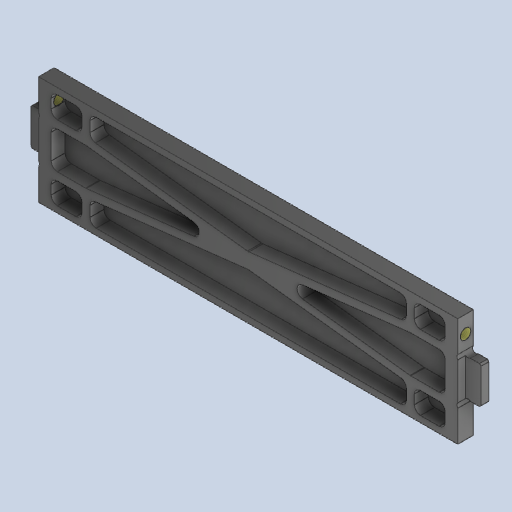
# Autodesk Inventor part: Cockpit_battery_front_frame
Saved by Autodesk Inventor 2022 (Build 260153000, 153)
## iProperties
Part Number: Cockpit_battery_front_frame
Material: アセタール樹脂、黒
Document SubType Name: Modeling
Designer: Masato Kubotera
Density: 1.425 g/cm^3
Appearance: 滑らか - 黒
Description: POM T5
Mass: 13.79 g
Surface Area: 149.623 cm^2
Volume: 9.6772 cm^3
Author: Masato Kubotera
Autodesk Inventor part; units mm, degrees
ref_plane "XZ Plane" through (0, 0, 0) normal (0, 1, 0) x (-1, 0, 0)
derived "Cockpit_side_frame.ipt"
sketch "スケッチ2" plane through (0, 0, 0) normal (0, 1, 0) x (-1, 0, 0)
  line L0 (-23.5, -22.5) -> (-28.5, -27.5)
  line L1 (-28.5, -27.5) -> (-28.5, -91)
  line L2 (-28.5, -91) -> (-23.5, -96)
  line L3 (-23.5, -96) -> (34.25, -96)
  line L4 (36.25, -98) -> (36.25, -131)
  line L5 (36.25, -131) -> (41.25, -136)
  line L6 (41.25, -136) -> (86.5, -136)
  line L7 (91.5, -131) -> (91.5, -20)
  line L8 (91.5, -20) -> (89, -17.5)
  line L9 (89, -17.5) -> (83.25, -17.5)
  line L10 (83.25, -17.5) -> (83.25, -21.0151)
  line L11 (81.7651, -22.5) -> (76.9849, -22.5)
  line L12 (75.5, -21.0151) -> (75.5, -17.5)
  line L13 (75.5, -17.5) -> (67.5, -17.5)
  line L14 (67.5, -17.5) -> (67.5, -21.0151)
  line L15 (66.0151, -22.5) -> (-23.5, -22.5)
  line L16 (-25.25, -25) -> (-20.25, -25) construction
  line L17 (-20.25, -25) -> (-20.25, -93.5) construction
  line L18 (-20.25, -93.5) -> (-25.25, -93.5) construction
  line L19 (-25.25, -93.5) -> (-25.25, -25) construction
  line L20 (-26, -25) -> (-25.25, -25) construction
  line L21 (-25.25, -93.5) -> (-26, -93.5) construction
  line L22 (-26, -93.5) -> (-26, -25) construction
  line L23 (-20.25, -93.5) -> (83.25, -93.5) construction
  line L24 (-20.25, -88.5) -> (83.25, -88.5) construction
  line L25 (83.25, -22.5) -> (83.25, -90.5) construction
  line L26 (83.25, -90.5) -> (88.25, -90.5) construction
  line L27 (88.25, -90.5) -> (88.25, -22.5) construction
  line L28 (83.25, -88.5) -> (83.25, -93.5) construction
  line L29 (83.25, -91) -> (88.25, -91) construction
  line L30 (88.25, -91) -> (88.25, -133.5) construction
  line L31 (83.25, -91) -> (83.25, -133.5) construction
  line L32 (83.25, -133.5) -> (88.25, -133.5) construction
  line L33 (38.75, -133.5) -> (38.75, -128.5) construction
  line L34 (38.75, -128.5) -> (38.75, -93.5) construction
  line L35 (43.75, -93.5) -> (43.75, -128.5) construction
  line L36 (38.75, -128.5) -> (43.75, -128.5) construction
  line L37 (41.25, -128.5) -> (41.25, -93.5) construction
  line L38 (38.75, -128.5) -> (82.1145, -128.5) construction
  line L39 (82.1145, -128.5) -> (82.1145, -133.5) construction
  line L40 (82.1145, -133.5) -> (38.75, -133.5) construction
  line L41 (38.75, -131) -> (82.1145, -131) construction
  line L42 (85.75, -91) -> (85.75, -133.5) construction
  circle A0 centre (85.75, -131) radius 2
  arc A1 (83.25, -128.5) -> (88.25, -128.5) centre (85.75, -131) ccw construction
  line L43 (83.25, -91) -> (-20.25, -91) construction
  line L44 (41.25, -111) -> (43.75, -111) construction
  line L45 (60.4322, -128.5) -> (60.4322, -131) construction
  line L46 (41.2, -115.5651) -> (41.2, -106.4349)
  line L47 (43.8, -107.05) -> (43.8, -114.95)
  line L48 (43.8, -117.05) -> (41.2, -104.95) construction
  line L49 (41.2, -117.05) -> (43.8, -104.95) construction
  line L50 (56.4822, -128.45) -> (64.3822, -128.45)
  line L51 (64.9973, -131.05) -> (55.8672, -131.05)
  line L52 (54.3822, -128.45) -> (66.4822, -131.05) construction
  line L53 (66.4822, -128.45) -> (54.3822, -131.05) construction
  line L54 (41.25, -105) -> (43.75, -105) construction
  line L55 (41.25, -117) -> (43.75, -117) construction
  arc A2 (42.6849, -104.95) -> (41.2, -106.4349) centre (41.9425, -105.6925) ccw
  arc A3 (43.8, -107.05) -> (43.8, -104.95) centre (43.8, -106) ccw
  arc A4 (41.2, -115.5651) -> (42.6849, -117.05) centre (41.9425, -116.3075) ccw
  arc A5 (43.8, -117.05) -> (43.8, -114.95) centre (43.8, -116) ccw
  line L56 (54.4322, -131) -> (54.4322, -128.5) construction
  line L57 (66.4322, -128.5) -> (66.4322, -131) construction
  arc A6 (54.3822, -129.5651) -> (55.8672, -131.05) centre (55.1247, -130.3075) ccw
  arc A7 (56.4822, -128.45) -> (54.3822, -128.45) centre (55.4322, -128.45) ccw
  arc A8 (64.9973, -131.05) -> (66.4822, -129.5651) centre (65.7398, -130.3075) ccw
  arc A9 (66.4822, -128.45) -> (64.3822, -128.45) centre (65.4322, -128.45) ccw
  line L58 (54.3822, -129.5651) -> (54.3822, -128.45)
  line L59 (66.4822, -128.45) -> (66.4822, -129.5651)
  line L60 (42.6849, -104.95) -> (43.8, -104.95)
  line L61 (43.8, -117.05) -> (42.6849, -117.05)
  circle A10 centre (48.4322, -131) radius 1.6
  line L62 (88.25, -22.5) -> (88.25, -17.5) construction
  line L63 (89, -17.5) -> (89, -90.5) construction
  line L64 (89, -90.5) -> (88.25, -90.5) construction
  line L65 (-13.5, -82.5) -> (-13.5, -61)
  arc A11 (-13.5, -82.5) -> (-11.5, -84.5) centre (-11.5, -82.5) ccw
  line L66 (45.5, -84.5) -> (-11.5, -84.5)
  arc A12 (45.5, -84.5) -> (47.5, -82.5) centre (45.5, -82.5) ccw
  line L67 (47.5, -61) -> (47.5, -82.5)
  arc A13 (47.5, -61) -> (45.5, -59) centre (45.5, -61) ccw
  line L68 (-11.5, -59) -> (45.5, -59)
  arc A14 (-11.5, -59) -> (-13.5, -61) centre (-11.5, -61) ccw
  line L69 (31.5, -88.5) -> (31.5, -91) construction
  line L70 (85.75, -22.5) -> (85.75, -90.5) construction
  circle A15 centre (85.75, -34) radius 1.6
  circle A16 centre (85.75, -34) radius 3
  circle A17 centre (85.75, -79) radius 3
  circle A18 centre (85.75, -79) radius 1.6
  line L71 (88.25, -22.5) -> (83.25, -22.5) construction
  arc A19 (88.25, -91) -> (83.25, -91) centre (85.75, -131) ccw construction
  circle A20 centre (48.4322, -131) radius 3
  circle A21 centre (41.25, -99) radius 1.6
  circle A22 centre (41.25, -99) radius 3
  line L72 (6.5, -88.5) -> (6.5, -91) construction
  line L73 (56.5, -88.5) -> (56.5, -91) construction
  line L74 (55.0651, -91.05) -> (7.9349, -91.05)
  line L75 (6.45, -89.5651) -> (6.45, -88.45)
  line L76 (8.55, -88.45) -> (54.45, -88.45)
  line L77 (56.55, -88.45) -> (56.55, -89.5651)
  line L78 (56.55, -91.05) -> (6.45, -88.45) construction
  line L79 (6.45, -91.05) -> (56.55, -88.45) construction
  arc A23 (8.55, -88.45) -> (6.45, -88.45) centre (7.5, -88.45) ccw
  arc A24 (6.45, -89.5651) -> (7.9349, -91.05) centre (7.1925, -90.3075) ccw
  arc A25 (55.0651, -91.05) -> (56.55, -89.5651) centre (55.8075, -90.3075) ccw
  arc A26 (56.55, -88.45) -> (54.45, -88.45) centre (55.5, -88.45) ccw
  line L80 (-20.25, -41) -> (83.25, -41) construction
  line L81 (83.25, -36) -> (-20.25, -36) construction
  line L82 (-20.25, -36) -> (-20.25, -41) construction
  line L83 (-20.25, -38.5) -> (83.25, -38.5) construction
  line L84 (31.5, -41) -> (31.5, -36) construction
  line L85 (55.0651, -35.95) -> (7.9349, -35.95)
  line L86 (7.9349, -41.05) -> (55.0651, -41.05)
  line L87 (56.55, -35.95) -> (6.45, -41.05) construction
  line L88 (6.45, -35.95) -> (55.5877, -40.952) construction
  arc A27 (7.9349, -35.95) -> (6.45, -37.4349) centre (7.1925, -36.6925) ccw
  arc A28 (6.45, -39.5651) -> (7.9349, -41.05) centre (7.1925, -40.3075) ccw
  arc A29 (56.55, -37.4349) -> (55.0651, -35.95) centre (55.8075, -36.6925) ccw
  arc A30 (55.0651, -41.05) -> (56.55, -39.5651) centre (55.8075, -40.3075) ccw
  line L89 (6.5, -41) -> (6.5, -36) construction
  line L90 (56.5, -36) -> (56.5, -41) construction
  line L91 (6.45, -37.4349) -> (6.45, -39.5651)
  line L92 (56.55, -39.5651) -> (56.55, -37.4349)
  circle A31 centre (-1, -38.5) radius 1.6
  circle A32 centre (-1, -38.5) radius 3
  circle A33 centre (64, -38.5) radius 1.6
  circle A34 centre (64, -38.5) radius 3
  line L93 (-25.25, -49.25) -> (-26, -49.25) construction
  line L94 (-25.25, -69.25) -> (-26, -69.25) construction
  line L95 (-26, -59.25) -> (-25.25, -59.25) construction
  line L96 (-22.75, -25) -> (-22.75, -93.5) construction
  arc A35 (66.0151, -22.5) -> (67.5, -21.0151) centre (66.7575, -21.7575) ccw
  arc A36 (75.5, -21.0151) -> (76.9849, -22.5) centre (76.2425, -21.7575) ccw
  line L97 (59.75, -22.5) -> (59.75, -32.5) construction
  line L98 (59.75, -32.5) -> (83.25, -32.5) construction
  line L99 (83.25, -32.5) -> (83.25, -22.5) construction
  line L100 (71.5, -17.5) -> (71.5, -32.5) construction
  line L101 (63.5, -22.5) -> (63.5, -17.5) construction
  line L102 (79.5, -22.5) -> (79.5, -17.5) construction
  circle A37 centre (-22.75, -31.75) radius 1.6
  circle A38 centre (-22.75, -31.75) radius 3
  circle A39 centre (-22.75, -86.75) radius 1.6
  circle A40 centre (-22.75, -86.75) radius 3
  line L103 (67.5, -22.5) -> (75.5, -22.5)
  line L104 (88.25, -17.5) -> (52.5, -17.5) construction
  line L105 (52.5, -17.5) -> (52.5, -22.5) construction
  circle A41 centre (85.75, -98.5) radius 1.475
  circle A42 centre (85.75, -103.5) radius 1.475
  circle A43 centre (85.75, -108.5) radius 1.475
  line L106 (48.25, -93.5) -> (78.75, -93.5)
  line L107 (80.75, -95.5) -> (80.75, -124)
  line L108 (78.75, -126) -> (48.25, -126)
  line L109 (46.25, -124) -> (46.25, -95.5)
  arc A44 (48.25, -93.5) -> (46.25, -95.5) centre (48.25, -95.5) ccw
  arc A45 (46.25, -124) -> (48.25, -126) centre (48.25, -124) ccw
  arc A46 (78.75, -126) -> (80.75, -124) centre (78.75, -124) ccw
  arc A47 (80.75, -95.5) -> (78.75, -93.5) centre (78.75, -95.5) ccw
  arc A48 (36.25, -98) -> (34.25, -96) centre (34.25, -98) ccw
  circle A49 centre (-13.5, -55) radius 1.75
  circle A50 centre (-13.5, -55) radius 2
  line L110 (77.85, -78.65) -> (68.65, -78.65) construction
  line L111 (68.65, -78.65) -> (68.65, -64.85) construction
  line L112 (68.65, -64.85) -> (77.85, -64.85) construction
  line L113 (77.85, -64.85) -> (77.85, -78.65) construction
  line L114 (77.85, -78.65) -> (68.65, -64.85) construction
  line L115 (68.65, -78.65) -> (77.85, -64.85) construction
  line L116 (67.95, -64.2) -> (78.55, -64.2) construction
  line L117 (78.55, -64.2) -> (78.55, -79.3) construction
  line L118 (78.55, -79.3) -> (67.95, -79.3) construction
  line L119 (67.95, -79.3) -> (67.95, -64.2) construction
  line L120 (67.95, -64.2) -> (78.55, -79.3) construction
  line L121 (78.55, -64.2) -> (67.95, -79.3) construction
  line L122 (69.3849, -64.15) -> (77.1151, -64.15)
  line L123 (78.6, -65.6349) -> (78.6, -77.8651)
  line L124 (78.6, -79.35) -> (67.9, -64.15) construction
  line L125 (67.9, -79.35) -> (78.6, -64.15) construction
  line L126 (77.9, -78.7) -> (68.6, -64.8) construction
  line L127 (68.6, -78.7) -> (77.9, -64.8) construction
  arc A51 (69.3849, -64.15) -> (67.9, -65.6349) centre (68.6425, -64.8925) ccw
  arc A52 (70.0849, -64.8) -> (68.6, -66.2849) centre (69.3425, -65.5425) ccw
  line L128 (67.9, -71.75) -> (78.6, -71.75) construction
  line L129 (73.25, -64.15) -> (73.25, -78.7063) construction
  arc A53 (78.6, -65.6349) -> (77.1151, -64.15) centre (77.8575, -64.8925) ccw
  arc A54 (77.9, -66.2849) -> (76.4151, -64.8) centre (77.1575, -65.5425) ccw
  arc A55 (68.6, -77.2151) -> (70.0849, -78.7) centre (69.3425, -77.9575) ccw
  arc A56 (67.9, -77.8651) -> (69.3849, -79.35) centre (68.6425, -78.6075) ccw
  arc A57 (76.4151, -78.7) -> (77.9, -77.2151) centre (77.1575, -77.9575) ccw
  arc A58 (77.1151, -79.35) -> (78.6, -77.8651) centre (77.8575, -78.6075) ccw
  line L130 (70.0849, -64.8) -> (76.4151, -64.8)
  line L131 (77.9, -66.2849) -> (77.9, -77.2151)
  line L132 (67.9, -77.8651) -> (67.9, -65.6349)
  line L133 (68.6, -77.2151) -> (68.6, -66.2849)
  line L134 (76.4151, -78.7) -> (70.0849, -78.7)
  line L135 (77.1151, -79.35) -> (69.3849, -79.35)
  line L136 (-13.5, -71.75) -> (47.5, -71.75) construction
  line L137 (85.75, -56.5) -> (88.25, -56.5) construction
  line L138 (89, -54) -> (88.25, -54) construction
  line L139 (85.7, -69.45) -> (85.7, -43.55)
  line L140 (88.2835, -71.3588) -> (85.7, -41.45) construction
  line L141 (85.7, -71.55) -> (88.3, -41.45) construction
  arc A59 (85.7, -41.45) -> (85.7, -43.55) centre (85.7, -42.5) ccw
  arc A60 (88.3, -42.9349) -> (86.8151, -41.45) centre (87.5575, -42.1925) ccw
  arc A61 (85.7, -69.45) -> (85.7, -71.55) centre (85.7, -70.5) ccw
  arc A62 (86.8151, -71.55) -> (88.3, -70.0651) centre (87.5575, -70.8075) ccw
  line L142 (85.75, -41.5) -> (88.25, -41.5) construction
  line L143 (85.75, -71.5) -> (88.25, -71.5) construction
  arc A63 (89.25, -47.1801) -> (88.3, -46.1348) centre (88.2, -47.1801) ccw
  line L144 (89.25, -47.1801) -> (89.25, -65.8199)
  line L145 (88.25, -46.5) -> (89, -46.5) construction
  line L146 (88.25, -66.5) -> (89, -66.5) construction
  arc A64 (88.3, -66.8652) -> (89.25, -65.8199) centre (88.2, -65.8199) ccw
  line L147 (88.3, -42.9349) -> (88.3, -46.1348)
  line L148 (88.3, -66.8652) -> (88.3, -70.0651)
  line L149 (86.8151, -71.55) -> (85.7, -71.55)
  line L150 (85.7, -41.45) -> (86.8151, -41.45)
  line L151 (86.5, -136) -> (91.5, -131)
  arc A65 (81.7651, -22.5) -> (83.25, -21.0151) centre (82.5075, -21.7575) ccw
  circle A66 centre (85.75, -93.5) radius 2
  circle A67 centre (85.75, -93.5) radius 4 construction
  arc A68 (-24.15, -49.25) -> (-26.25, -49.25) centre (-25.2, -49.25) ccw
  line L152 (-26, -49.25) -> (-26.25, -49.25) construction
  line L153 (-26.25, -49.25) -> (-26.25, -69.25)
  line L154 (-24.15, -49.25) -> (-24.15, -69.25)
  arc A69 (-26.25, -69.25) -> (-24.15, -69.25) centre (-25.2, -69.25) ccw
  point P0 (0, 0)
  point P1 (-25.7227, -96)
  point P2 (-23.5, -22.5)
  point P3 (42.5, -111)
  point P4 (60.4322, -129.75)
  point P5 (31.5, -89.75)
  point P6 (31.5, -38.5)
  point P7 (6.45, -41.05)
  point P8 (52.5, -22)
  point P9 (73.25, -71.75)
  point P10 (73.25, -71.75)
  point P11 (87, -56.5)
  dimension "d1" = 43.75
  dimension "d2" = 5
  dimension "d3" = 2.5
  measures "d1" distance from line of point (0, 0) L35
  measures "d2" distance of L35.end L33.end
  measures "d3" distance of L55.start L55.end
ref_plane "作業平面1" through (-43.75, 0, 0) normal (1, 0, 0) x (0, 1, 0)
sketch "スケッチ3" plane through (-43.75, 0, 0) normal (1, 0, 0) x (0, 1, 0)
  line L0 (-135, -93.5) -> (0, -93.5)
  line L1 (0, -128.5) -> (-135, -128.5)
  line L2 (1.4849, -105) -> (5, -105)
  line L3 (5, -105) -> (5, -117)
  arc A0 (0, -103.5151) -> (1.4849, -105) centre (0.7425, -104.2575) ccw
  line L4 (0, -93.5) -> (0, -103.5151)
  line L5 (-134.9908, -111) -> (0, -111) construction
  line L6 (1.4849, -117) -> (5, -117)
  arc A1 (1.4849, -117) -> (0, -118.4849) centre (0.7425, -117.7425) ccw
  line L7 (0, -128.5) -> (0, -118.4849)
  line L8 (0, -105) -> (0, -117)
  line L9 (0, -118.4849) -> (0, -128.5)
  line L10 (-67.5, -93.5) -> (-67.5, -128.5) construction
  line L11 (-136.4849, -105) -> (-140, -105)
  line L12 (-140, -105) -> (-140, -117)
  arc A2 (-136.4849, -105) -> (-135, -103.5151) centre (-135.7425, -104.2575) ccw
  line L13 (-135, -93.5) -> (-135, -103.5151)
  line L14 (-136.4849, -117) -> (-140, -117)
  arc A3 (-135, -118.4849) -> (-136.4849, -117) centre (-135.7425, -117.7425) ccw
  line L15 (-135, -128.5) -> (-135, -118.4849)
  line L16 (-135, -105) -> (-135, -117)
  line L17 (-135, -118.4849) -> (-135, -128.5)
  line L18 (-12, -119.5) -> (-6, -119.5)
  line L19 (-4, -121.5) -> (-4, -124.5)
  line L20 (-6, -126.5) -> (-12, -126.5)
  line L21 (-14, -124.5) -> (-14, -121.5)
  line L22 (-4, -115) -> (-4, -107)
  line L23 (-67.2707, -113.5132) -> (-18.2707, -119.168)
  line L24 (-16.5, -121.1548) -> (-16.5, -124.5)
  line L25 (-18.5, -126.5) -> (-116.5, -126.5)
  line L26 (-6, -117) -> (-15.135, -117)
  line L27 (-15.3643, -116.9868) -> (-50.0251, -112.9868)
  line L28 (-12, -102.5) -> (-6, -102.5)
  line L29 (-4, -100.5) -> (-4, -97.5)
  line L30 (-6, -95.5) -> (-12, -95.5)
  line L31 (-14, -97.5) -> (-14, -100.5)
  line L32 (-67.2707, -108.4868) -> (-18.2707, -102.832)
  line L33 (-16.5, -100.8452) -> (-16.5, -97.5)
  line L34 (-18.5, -95.5) -> (-116.5, -95.5)
  line L35 (-6, -105) -> (-15.135, -105)
  line L36 (-15.3643, -105.0132) -> (-50.0251, -109.0132)
  line L37 (-67.7293, -113.5132) -> (-116.7293, -119.168)
  line L38 (-118.5, -121.1548) -> (-118.5, -124.5)
  line L39 (-118.5, -100.8452) -> (-118.5, -97.5)
  line L40 (-67.7293, -108.4868) -> (-116.7293, -102.832)
  arc A4 (-6, -126.5) -> (-4, -124.5) centre (-6, -124.5) ccw
  arc A5 (-4, -121.5) -> (-6, -119.5) centre (-6, -121.5) ccw
  arc A6 (-12, -119.5) -> (-14, -121.5) centre (-12, -121.5) ccw
  arc A7 (-14, -124.5) -> (-12, -126.5) centre (-12, -124.5) ccw
  arc A8 (-18.5, -126.5) -> (-16.5, -124.5) centre (-18.5, -124.5) ccw
  arc A9 (-16.5, -121.1548) -> (-18.2707, -119.168) centre (-18.5, -121.1548) ccw
  arc A10 (-67.2707, -113.5132) -> (-67.7293, -113.5132) centre (-67.5, -115.5) ccw
  arc A11 (-116.7293, -119.168) -> (-118.5, -121.1548) centre (-116.5, -121.1548) ccw
  arc A12 (-118.5, -124.5) -> (-116.5, -126.5) centre (-116.5, -124.5) ccw
  arc A13 (-118.5, -100.8452) -> (-116.7293, -102.832) centre (-116.5, -100.8452) ccw
  arc A14 (-116.5, -95.5) -> (-118.5, -97.5) centre (-116.5, -97.5) ccw
  arc A15 (-16.5, -97.5) -> (-18.5, -95.5) centre (-18.5, -97.5) ccw
  arc A16 (-18.2707, -102.832) -> (-16.5, -100.8452) centre (-18.5, -100.8452) ccw
  arc A17 (-67.7293, -108.4868) -> (-67.2707, -108.4868) centre (-67.5, -106.5) ccw
  arc A18 (-50.0251, -109.0132) -> (-50.0251, -112.9868) centre (-49.7958, -111) ccw
  arc A19 (-15.135, -105) -> (-15.3643, -105.0132) centre (-15.135, -107) ccw
  arc A20 (-4, -107) -> (-6, -105) centre (-6, -107) ccw
  arc A21 (-6, -117) -> (-4, -115) centre (-6, -115) ccw
  arc A22 (-15.3643, -116.9868) -> (-15.135, -117) centre (-15.135, -115) ccw
  arc A23 (-14, -100.5) -> (-12, -102.5) centre (-12, -100.5) ccw
  arc A24 (-12, -95.5) -> (-14, -97.5) centre (-12, -97.5) ccw
  arc A25 (-4, -97.5) -> (-6, -95.5) centre (-6, -97.5) ccw
  arc A26 (-6, -102.5) -> (-4, -100.5) centre (-6, -100.5) ccw
  line L41 (-123, -119.5) -> (-129, -119.5)
  line L42 (-121, -124.5) -> (-121, -121.5)
  line L43 (-131, -115) -> (-131, -107)
  line L44 (-129, -117) -> (-119.865, -117)
  line L45 (-119.6357, -116.9868) -> (-84.9749, -112.9868)
  line L46 (-123, -102.5) -> (-129, -102.5)
  line L47 (-121, -97.5) -> (-121, -100.5)
  line L48 (-129, -95.5) -> (-123, -95.5)
  line L49 (-131, -100.5) -> (-131, -97.5)
  line L50 (-119.6357, -105.0132) -> (-84.9749, -109.0132)
  line L51 (-129, -105) -> (-119.865, -105)
  arc A27 (-131, -124.5) -> (-129, -126.5) centre (-129, -124.5) ccw
  arc A28 (-129, -119.5) -> (-131, -121.5) centre (-129, -121.5) ccw
  arc A29 (-121, -121.5) -> (-123, -119.5) centre (-123, -121.5) ccw
  arc A30 (-123, -126.5) -> (-121, -124.5) centre (-123, -124.5) ccw
  arc A31 (-84.9749, -112.9868) -> (-84.9749, -109.0132) centre (-85.2042, -111) ccw
  arc A32 (-119.6357, -105.0132) -> (-119.865, -105) centre (-119.865, -107) ccw
  arc A33 (-129, -105) -> (-131, -107) centre (-129, -107) ccw
  arc A34 (-131, -115) -> (-129, -117) centre (-129, -115) ccw
  arc A35 (-119.865, -117) -> (-119.6357, -116.9868) centre (-119.865, -115) ccw
  arc A36 (-123, -102.5) -> (-121, -100.5) centre (-123, -100.5) ccw
  arc A37 (-121, -97.5) -> (-123, -95.5) centre (-123, -97.5) ccw
  arc A38 (-129, -95.5) -> (-131, -97.5) centre (-129, -97.5) ccw
  arc A39 (-131, -100.5) -> (-129, -102.5) centre (-129, -100.5) ccw
  line L52 (-129, -126.5) -> (-123, -126.5)
  line L53 (-4, -99) -> (0, -99) construction
  line L54 (-131, -121.5) -> (-131, -124.5)
  point P0 (0, 0)
  point P1 (0, -128.5)
  point P2 (-135, -111)
  point P3 (-14, -119.5)
  point P4 (-4, -126.5)
  point P5 (-4, -119.5)
  point P6 (-14, -126.5)
  point P7 (-4, -117)
  point P8 (-67.5, -113.4867)
  point P9 (-16.5, -119.3723)
  point P10 (-16.5, -126.5)
  point P11 (-118.5, -126.5)
  point P12 (-15.25, -117)
  point P13 (-67.2412, -111)
  point P14 (-14, -102.5)
  point P15 (-4, -95.5)
  point P16 (-4, -102.5)
  point P17 (-14, -95.5)
  point P18 (-4, -105)
  point P19 (-67.5, -108.5133)
  point P20 (-16.5, -102.6277)
  point P21 (-16.5, -95.5)
  point P22 (-15.25, -105)
  point P23 (-118.5, -119.3723)
  point P24 (-118.5, -126.5)
  point P25 (-118.5, -102.6277)
  point P26 (-118.5, -95.5)
  dimension "d5" = 5
  dimension "d6" = 135
  dimension "d7" = 1.05
  dimension "d19" = 4
  dimension "d20" = 2
  dimension "d21" = 10
  dimension "d22" = 2.5
  dimension "d23" = 11.25
  dimension "d24" = 2.5
  dimension "d25" = 2
  dimension "d26" = 2.5
  dimension "d27" = 5
  constraints: 110 end point, 85 point on circle, 72 symmetric about line, 58 point on line, 46 tangent, 40 centre point, 22 equal radius, 9 perpendicular, 5 midpoint, 5 parallel, 4 horizontal, 3 coincident, 2 collinear, 1 vertical, 16 other
  measures "d5" distance between parallel lines of L3 L8
  measures "d6" distance of L0.start L0.end
  measures "d7" radius of A0
  measures "d19" distance between parallel lines of L7 L19
  measures "d20" distance between parallel lines of L1 L20
  measures "d21" distance of point (-4, -126.5) point (-14, -126.5)
  measures "d22" distance between parallel lines of L24 L21
  measures "d23" distance of point (-4, -117) point (-15.25, -117)
  measures "d24" distance between parallel lines of L23 L27
  measures "d25" radius of A4
  measures "d26" distance between parallel lines of L18 L26
extrude "押し出し1" add sketch "スケッチ3" along normal blind 5 contours L0 L4 A0 L8 A1 L7 L1 L15 A3 L16 A2 L13
extrude "押し出し2" add sketch "スケッチ3" along normal blind 2.5 contours L16 A3 L14 L12 L11 A2 | A0 L2 L3 L6 A1 L8
hole "穴1" at (-41.25, 0, -99) direction (0, -1, 0) diameter 3.4587 depth 4 thread size "M4x0.5" class "6H" standard "ANSI Metric M Profile"
ref_plane "作業平面2" through (-43.75, -67.5, -93.5) normal (0, 1, 0) x (1, 0, 0)
mirror "ミラー1" about plane through (-43.75, -67.5, -93.5) normal (0, 1, 0) of "穴1"
extrude "押し出し3" add sketch "スケッチ3" along normal blind 0.5 contours L18 A5 L19 A4 L20 A7 L21 A6 | A21 L26 A22 L27 A18 L36 A19 L35 A20 L22 | L23 A9 L24 A8 L25 A12 L38 A11 L37 A10 | A23 L31 A24 L30 A25 L29 A26 L28 | A17 L40 A13 L39 A14 L34 A15 L33 A16 L32 | A29 L42 A30 L52 A27 L54 A28 L41 | L43 A33 L51 A32 L50 A31 L45 A35 L44 A34 | L46 A39 L49 A38 L48 A37 L47 A36
chamfer "面取り1" distance 0.5 angle 45 4 edges at (-42.5, -140, -117) (-42.5, -140, -105) (-42.5, 5, -117) (-42.5, 5, -105)
equation "\"d23\" = d21 + 0.5 * d22"
equation "\"d24\" = d22"
equation "\"d26\" = d22"
equation "\"d27\" = 2 * d22"
equation "\"d8\" = d2"
equation "\"d10\" = d3"
equation "\"d4\" = -d1"
